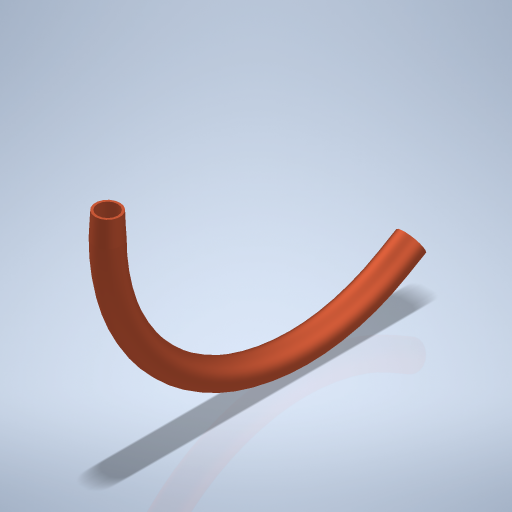
# Autodesk Inventor part: Tube
Saved by Autodesk Inventor 2024 (Build 280153000, 153)
## iProperties
Created: 2024-06-06
Part Number: Tube
Material: Kupfer
Document SubType Name: Modeling
Designer: ffogue
Density: 8.94 g/cm^3
Appearance: Kupfer - satiniert
Author: ffogue
Autodesk Inventor part; units mm, degrees
ref_plane "YZ Plane" through (0, 0, 0) normal (1, 0, 0) x (0, 1, 0)
sketch "Skizze1" plane through (0, 0, 0) normal (0, 0, 1) x (0, 1, 0)
  circle A0 centre (0, 0) radius 2.75
  dimension "d0" = 5.5
  constraints: 1 centre point, 1 coincident
  measures "d0" diameter of A0
sketch "Skizze2" plane through (0, 0, 0) normal (1, 0, 0) x (0, 1, 0)
  arc A0 (0, -5.5) -> (63.45, -42.1329) centre (42.3, -5.5) ccw
  line L0 (63.45, -42.1329) -> (67.5203, -39.7829)
  line L1 (42.3, -5.5) -> (42.3, -47.8) construction
  point P0 (0, 0)
  point P1 (0, 0)
  dimension "d3" = 5.5
  dimension "d4" = 42.3
  dimension "d5" = 4.7
  dimension "d27" = 60
  constraints: 4 end point, 3 point on circle, 1 centre point, 1 tangent, 1 vertical, 1 vertical alignment
  measures "d3" distance of point (0, 0) A0.start
  measures "d4" radius of A0
  measures "d5" distance of L0.start L0.end
  measures "d27" angle of L1 L0
ref_plane "Arbeitsebene1" through (0, 0, -5.5) normal (0, 0, 1) x (1, 0, 0)
sketch "Skizze3" plane through (0, 0, -5.5) normal (0, 0, 1) x (1, 0, 0)
  circle A0 centre (0, 0) radius 3
  dimension "d11" = 6
  constraints: 1 centre point, 1 coincident
  measures "d11" diameter of A0
ref_plane "Arbeitsebene2" through (0, 0, -5.5) normal (0, 0, -1) x (-1, 0, 0)
sketch "Skizze4" plane through (0, 0, -5.5) normal (0, 0, -1) x (-1, 0, 0)
  circle A0 centre (0, 0) radius 3 projected
loft "Erhebung2" add profiles "Skizze1", "Skizze3"
sweep "Sweeping3" add profiles "Skizze4" path "Skizze2"
shell "Wandung2" thickness 0.5 removed faces 2 at (-0.6079, 0.6861, 0) at (-0.7485, 67.8519, -40.3572)
